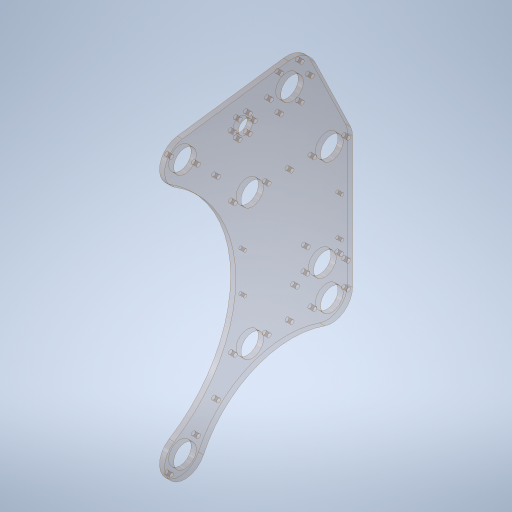
# Autodesk Inventor part: GP5-003
Saved by Autodesk Inventor 2023.4 (Build 274418000, 418)
## iProperties
Created: 2025-02-03
Part Number: GP5-003
Material: Polycarbonate, Smoke
Document SubType Name: Modeling
Designer: slick
Density: 1.2 g/cm^3
Appearance: Polycarbonate - Smoked
Mass: 361.739 g
Surface Area: 1106.19 cm^2
Volume: 301.449 cm^3
Author: slick
Autodesk Inventor part; units mm, degrees
ref_plane "YZ Plane" through (0, 0, 0) normal (1, 0, 0) x (0, 1, 0)
ref_plane "XZ Plane" through (0, 0, 0) normal (0, 1, 0) x (-1, 0, 0)
ref_plane "XY Plane" through (0, 0, 0) normal (0, 0, 1) x (1, 0, 0)
sketch "Sketch1" plane through (0, 0, 0) normal (1, 0, 0) x (0, 1, 0)
  line L0 (-12.7, 25.4) -> (12.7, 25.4) construction
  line L1 (12.7, 25.4) -> (12.7, -25.4) construction
  line L2 (12.7, -25.4) -> (-12.7, -25.4) construction
  line L3 (-12.7, -25.4) -> (-12.7, 25.4) construction
  line L4 (-12.7, 25.4) -> (12.7, -25.4) construction
  line L5 (12.7, 25.4) -> (-12.7, -25.4) construction
  circle A0 centre (-127, -49.4995) radius 38.1 construction
  circle A1 centre (-290.4981, -49.4995) radius 38.1 construction
  circle A2 centre (-127, 49.4995) radius 38.1 construction
  circle A3 centre (-290.4981, 49.4995) radius 38.1 construction
  line L6 (-127, -49.4995) -> (-127, 49.4995) construction
  line L7 (-290.4981, -49.4995) -> (-290.4981, 49.4995) construction
  line L8 (-161.925, -152.4) -> (-255.5731, -152.4) construction
  line L9 (-255.5731, -152.4) -> (-255.5731, 152.4) construction
  line L10 (-255.5731, 152.4) -> (-161.925, 152.4) construction
  line L11 (-161.925, 152.4) -> (-161.925, -152.4) construction
  line L12 (-161.925, -152.4) -> (-255.5731, 152.4) construction
  line L13 (-255.5731, -152.4) -> (-161.925, 152.4) construction
  circle A4 centre (-127, -49.4995) radius 34.925 construction
  circle A5 centre (-290.4981, -49.4995) radius 34.925 construction
  circle A6 centre (-208.749, 279.4) radius 190.5 construction
  circle A7 centre (-49.7545, 133.3399) radius 25.4 construction
  circle A8 centre (-367.7435, 133.3399) radius 25.4 construction
  circle A9 centre (-653.2508, -157.862) radius 53.975 construction
  line L14 (-596.1008, -277.7111) -> (-621.5008, -277.7111) construction
  line L15 (-621.5008, -277.7111) -> (-621.5008, -201.5111) construction
  line L16 (-621.5008, -201.5111) -> (-596.1008, -201.5111) construction
  line L17 (-596.1008, -201.5111) -> (-596.1008, -277.7111) construction
  line L18 (-596.1008, -277.7111) -> (-621.5008, -201.5111) construction
  line L19 (-621.5008, -277.7111) -> (-596.1008, -201.5111) construction
  line L20 (-685.0008, -277.7111) -> (-710.4008, -277.7111) construction
  line L21 (-710.4008, -277.7111) -> (-710.4008, -201.5111) construction
  line L22 (-710.4008, -201.5111) -> (-685.0008, -201.5111) construction
  line L23 (-685.0008, -201.5111) -> (-685.0008, -277.7111) construction
  line L24 (-685.0008, -277.7111) -> (-710.4008, -201.5111) construction
  line L25 (-710.4008, -277.7111) -> (-685.0008, -201.5111) construction
  line L26 (-498.4346, -157.862) -> (-808.067, -157.862) construction
  point P0 (0, 0)
  point P1 (-127, 0)
  point P2 (-290.4981, 0)
  point P3 (-208.749, 0)
  point P4 (-608.8008, -239.6111)
  point P5 (-697.7008, -239.6111)
  dimension "d0" = 25.4
  dimension "d1" = 50.8
  dimension "d2" = 76.2
  dimension "d4" = 98.999
  dimension "d5" = 93.6481
  dimension "d6" = 304.8
  dimension "d7" = 3.175
  dimension "d8" = 3.175
  dimension "d9" = 127
  dimension "d10" = 381
  dimension "d11" = 50.8
  dimension "d12" = 50.8
  dimension "d13" = 114.0003
  dimension "d14" = 279.4
  dimension "d35" = 49.4995
  dimension "d68" = 107.95
  dimension "d69" = 25.4
  dimension "d70" = 76.2
  dimension "d71" = 63.5
  dimension "d72" = 81.749
  dimension "d73" = 163.4981
  constraints: 54 end point, 11 midpoint, 10 centre point, 8 parallel, 7 horizontal alignment, 5 horizontal, 4 perpendicular, 4 tangent, 3 equal radius, 3 vertical alignment, 2 equal length, 2 point on circle, 2 vertical, 1 coincident
  measures "d0" distance of L1.end L2.end
  measures "d1" distance of L0.end L1.end
  measures "d2" diameter of A0
  measures "d4" distance of L6.start L6.end
  measures "d5" distance of L9.end L10.end
  measures "d6" distance of L8.end L9.end
  measures "d7" radial gap between concentric circles of A0 A4
  measures "d8" radial gap between concentric circles of A1 A5
  measures "d9" distance from line of point (0, 0) L6
  measures "d10" diameter of A6
  measures "d11" diameter of A7
  measures "d12" diameter of A8
  measures "d13" distance of L6.end A7.centre
  measures "d14" distance of A6.centre point (-208.749, 0)
  measures "d35" distance of L6.start point (-127, 0)
  measures "d68" diameter of A9
  measures "d69" distance of L15.end L16.end
  measures "d70" distance of L14.end L15.end
  measures "d71" distance of L20.start L14.end
  measures "d72" vertical distance of A9.centre point (-608.801, -239.611)
  measures "d73" distance of L7.start L6.start
sketch "Sketch2" plane through (0, 0, 0) normal (1, 0, 0) x (0, 1, 0)
  circle A0 centre (-127, -49.4995) radius 38.1 construction
  circle A1 centre (-127, 49.4995) radius 38.1 construction
  circle A2 centre (-127, -49.4995) radius 34.925 construction
  line L0 (-255.5731, 152.4) -> (-161.925, 152.4) construction
  line L1 (-161.925, -152.4) -> (-255.5731, -152.4) construction
  line L2 (-161.925, 152.4) -> (-161.925, -152.4) construction
  line L3 (-255.5731, -152.4) -> (-161.925, 152.4) construction
  line L4 (-161.925, -152.4) -> (-255.5731, 152.4) construction
  line L5 (-255.5731, -152.4) -> (-255.5731, 152.4) construction
  circle A3 centre (-290.4981, 49.4995) radius 38.1 construction
  circle A4 centre (-290.4981, -49.4995) radius 34.925 construction
  circle A5 centre (-290.4981, -49.4995) radius 38.1 construction
  line L6 (-290.4981, -49.4995) -> (-290.4981, 49.4995) construction
  line L7 (-127, -49.4995) -> (-127, 49.4995) construction
  line L8 (-12.7, -25.4) -> (-12.7, 25.4) construction
  line L9 (12.7, 25.4) -> (12.7, -25.4) construction
  line L10 (12.7, -25.4) -> (-12.7, -25.4) construction
  line L11 (-12.7, 25.4) -> (12.7, -25.4) construction
  line L12 (12.7, 25.4) -> (-12.7, -25.4) construction
  line L13 (-12.7, 25.4) -> (12.7, 25.4) construction
  circle A6 centre (-208.749, 279.4) radius 190.5 construction
  circle A7 centre (-49.7545, 133.3399) radius 25.4 construction
  circle A8 centre (-367.7435, 133.3399) radius 25.4 construction
  circle A9 centre (-127, -49.4995) radius 14.1605
  circle A10 centre (-290.4981, -49.4995) radius 14.1605
  circle A11 centre (-290.4981, 49.4995) radius 14.1605
  circle A12 centre (-127, 49.4995) radius 14.1605
  circle A13 centre (-367.7435, 133.3399) radius 14.1605
  circle A14 centre (-49.7545, 133.3399) radius 14.1605
  circle A15 centre (-38.1, 0) radius 14.1605
  circle A16 centre (-38.1, 0) radius 39.3065 construction
  circle A17 centre (-38.1, 0) radius 25.4 construction
  circle A18 centre (-38.1, 0) radius 31.75 construction
  circle A19 centre (-127, -49.4995) radius 25.781 construction
  line L14 (-127, -70.518) -> (-127, -28.481) construction
  circle A20 centre (-127, -70.518) radius 4.7625 construction
  circle A21 centre (-290.4981, -49.4995) radius 25.781 construction
  circle A22 centre (-290.4981, 49.4995) radius 25.781 construction
  circle A23 centre (-127, 49.4995) radius 25.781 construction
  line L15 (-127, -75.2805) -> (-290.4981, -75.2805)
  arc A24 (-314.7766, -40.827) -> (-378.357, 110.2636) centre (-429.0704, 0) ccw
  line L16 (-115.8012, -72.7212) -> (-24.3083, -28.5981)
  line L17 (-6.6374, 4.262) -> (-24.5844, 136.7495)
  arc A25 (-346.1366, 146.6928) -> (-71.3615, 146.6928) centre (-208.749, 231.5971) ccw
  arc A26 (-24.5844, 136.7495) -> (-71.3615, 146.6928) centre (-49.7545, 133.3399) ccw
  arc A27 (-346.1366, 146.6928) -> (-378.357, 110.2636) centre (-367.7435, 133.3399) ccw
  arc A28 (-314.7766, -40.827) -> (-290.4981, -75.2805) centre (-290.4981, -49.4995) ccw
  arc A29 (-127, -75.2805) -> (-115.8012, -72.7212) centre (-127, -49.4995) ccw
  arc A30 (-24.3083, -28.5981) -> (-6.6374, 4.262) centre (-38.1, 0) ccw
  circle A31 centre (-50.8, 58.2876) radius 19.05 construction
  circle A32 centre (-50.8, 58.2876) radius 12.7 construction
  circle A33 centre (-50.8, 58.2876) radius 8.763
  line L18 (-290.4981, 28.481) -> (-290.4981, 70.518) construction
  line L19 (-290.4981, -70.518) -> (-290.4981, -28.481) construction
  line L20 (-62.4545, 116.5921) -> (-37.0545, 150.0876) construction
  line L21 (-355.0435, 116.5921) -> (-380.4435, 150.0876) construction
  line L22 (-127, 28.481) -> (-127, 70.518) construction
  circle A34 centre (-248.1928, -40.8522) radius 14.1605
  circle A35 centre (-248.1928, -40.8522) radius 21.59 construction
  circle A36 centre (-290.4981, -49.4995) radius 21.59 construction
  line L23 (-248.1928, -61.8707) -> (-248.1928, -19.8337) construction
  point P0 (0, 0)
  point P1 (-127, 0)
  point P2 (-208.749, 0)
  point P3 (-290.4981, 0)
  point P4 (0, 0)
  point P5 (-38.1, 25.4)
  point P6 (-395.5081, 116.5261)
  point P7 (-50.8, 45.5876)
  point P8 (-39.8015, 51.9376)
  point P9 (-39.8015, 64.6376)
  point P10 (-50.8, 70.9876)
  point P11 (-61.7985, 64.6376)
  point P12 (-61.7985, 51.9376)
  dimension "d18" = 50.8
  dimension "d32" = 9.525
  dimension "d37" = 25.4
  dimension "d15" = 28.321
  dimension "d16" = 38.1
  dimension "d17" = 78.613
  dimension "d19" = 6.35
  dimension "d31" = 42.037
  dimension "d36" = 38.1
  dimension "d38" = 17.526
  dimension "d50" = 12.7
  dimension "d51" = 12.7
  dimension "d61" = 360
  dimension "d63" = 75.0595
  dimension "d64" = 76.2
  dimension "d74" = 121.5009
  dimension "d75" = 43.18
  constraints: 25 centre point, 25 coincident, 24 point on circle, 20 end point, 12 equal radius, 11 tangent, 10 vertical alignment, 7 midpoint, 6 equal length, 2 horizontal, 1 collinear, 1 horizontal alignment, 1 point on line, 14 other
  measures "d15" diameter of A9
  measures "d16" distance of A15.centre point (0, 0)
  measures "d17" diameter of A16
  measures "d31" distance of L14.end L14.start
  measures "d36" diameter of A31
  measures "d38" diameter of A33
  measures "d50" horizontal distance of point (-49.755, 133.34) L20.start
  measures "d51" horizontal distance of A8.centre L21.start
  measures "d63" distance of A7.centre A31.centre
  measures "d64" horizontal distance of L7.end A31.centre
  measures "d74" distance of A34.centre A0.centre
  measures "d75" diameter of A35
extrude "Extrusion1" add sketch "Sketch2" along normal blind 6.35
hole "Hole1" at (0, -127, -49.4995) at (0, -127, 49.4995) at (0, -161.925, 152.4) at (0, -161.925, -152.4) at (0, -255.5731, 152.4) at (0, -290.4981, 49.4995) at (0, -290.4981, -49.4995) at (0, -255.5731, -152.4) at (0, -127, -70.518) at (0, -127, -28.481) at (0, -50.8, 45.5876) at (0, -290.4981, 28.481) at (0, -290.4981, 70.518) at (0, -290.4981, -70.518) at (0, -290.4981, -28.481) at (0, -62.4545, 116.5921) at (0, -37.0545, 150.0876) at (0, -355.0435, 116.5921) at (0, -380.4435, 150.0876) at (0, -127, 28.481) at (0, -127, 70.518) at (0, -61.7985, 51.9376) at (0, -61.7985, 64.6376) at (0, -50.8, 70.9876) at (0, -39.8015, 64.6376) at (0, -39.8015, 51.9376) at (0, -248.1928, -61.8707) at (0, -248.1928, -19.8337) direction (1, 0, 0) diameter 5.1054 end through all clearance for "Flat Head Machine Screw (82)" size "#10" standard "Ansi Unified Screw Threads"
sketch "Sketch3" plane through (6.35, 0, 0) normal (1, 0, 0) x (0, 0, -1)
  circle A0 centre (0, -38.1) radius 14.1605 construction
  circle A1 centre (0, -38.1) radius 25.4 construction
  point P0 (0, 0)
  point P1 (25.4, -38.1)
  point P2 (12.7, -16.103)
  point P3 (-12.7, -16.103)
  point P4 (-25.4, -38.1)
  point P5 (-12.7, -60.097)
  point P6 (12.7, -60.097)
  dimension "d77" = 50.8
  dimension "d80" = 360
  constraints: 2 horizontal alignment, 1 coincident, 9 other
hole "Hole2" at (6.35, -38.1, -25.4) at (6.35, -16.103, -12.7) at (6.35, -16.103, 12.7) at (6.35, -38.1, 25.4) at (6.35, -60.097, 12.7) at (6.35, -60.097, -12.7) direction (-1, 0, 0) diameter 5.1054 end through all clearance for "Flat Head Machine Screw (82)" size "#10" standard "Ansi Unified Screw Threads"
sketch "Sketch4" plane through (6.35, 0, 0) normal (1, 0, 0) x (0, 0, -1)
  circle A0 centre (-12.7, -60.097) radius 2.5527 projected
  circle A1 centre (-12.7, -16.103) radius 2.5527 projected
  circle A2 centre (25.4, -38.1) radius 2.5527 projected
  circle A3 centre (12.7, -16.103) radius 2.5527 projected
  circle A4 centre (-25.4, -38.1) radius 2.5527 projected
  circle A5 centre (12.7, -60.097) radius 2.5527 projected
  circle A6 centre (61.8707, -248.1928) radius 2.5527 projected
  circle A7 centre (-64.6376, -39.8015) radius 2.5527 projected
  circle A8 centre (-64.6376, -61.7985) radius 2.5527 projected
  circle A9 centre (-70.518, -127) radius 2.5527 projected
  circle A10 centre (-150.0876, -380.4435) radius 2.5527 projected
  circle A11 centre (-150.0876, -37.0545) radius 2.5527 projected
  circle A12 centre (28.481, -290.4981) radius 2.5527 projected
  circle A13 centre (-70.518, -290.4981) radius 2.5527 projected
  circle A14 centre (-45.5876, -50.8) radius 2.5527 projected
  circle A15 centre (70.518, -127) radius 2.5527 projected
  circle A16 centre (28.481, -127) radius 2.5527 projected
  circle A17 centre (-28.481, -290.4981) radius 2.5527 projected
  circle A18 centre (70.518, -290.4981) radius 2.5527 projected
  circle A19 centre (-116.5921, -62.4545) radius 2.5527 projected
  circle A20 centre (-116.5921, -355.0435) radius 2.5527 projected
  circle A21 centre (-28.481, -127) radius 2.5527 projected
  circle A22 centre (-51.9376, -61.7985) radius 2.5527 projected
  circle A23 centre (-70.9876, -50.8) radius 2.5527 projected
  circle A24 centre (-51.9376, -39.8015) radius 2.5527 projected
  circle A25 centre (19.8337, -248.1928) radius 2.5527 projected
  arc A26 (28.5981, -24.3083) -> (-4.262, -6.6374) centre (0, -38.1) ccw projected
  line L0 (-4.262, -6.6374) -> (-136.7495, -24.5844) projected
  arc A27 (-136.7495, -24.5844) -> (-146.6928, -71.3615) centre (-133.3399, -49.7545) ccw projected
  arc A28 (-146.6928, -346.1366) -> (-146.6928, -71.3615) centre (-231.5971, -208.749) ccw projected
  arc A29 (-146.6928, -346.1366) -> (-110.2636, -378.357) centre (-133.3399, -367.7435) ccw projected
  arc A30 (40.827, -314.7766) -> (-110.2636, -378.357) centre (0, -429.0704) ccw projected
  arc A31 (40.827, -314.7766) -> (75.2805, -290.4981) centre (49.4995, -290.4981) ccw projected
  line L1 (75.2805, -290.4981) -> (75.2805, -127) projected
  arc A32 (75.2805, -127) -> (72.7212, -115.8012) centre (49.4995, -127) ccw projected
  line L2 (72.7212, -115.8012) -> (28.5981, -24.3083) projected
  circle A33 centre (-49.4995, -290.4981) radius 14.1605 projected
  circle A34 centre (-49.4995, -127) radius 14.1605 projected
  circle A35 centre (-58.2876, -50.8) radius 8.763 projected
  circle A36 centre (40.8522, -248.1928) radius 14.1605 projected
  circle A37 centre (0, -38.1) radius 14.1605 projected
  circle A38 centre (-133.3399, -49.7545) radius 14.1605 projected
  circle A39 centre (-133.3399, -367.7435) radius 14.1605 projected
  circle A40 centre (49.4995, -290.4981) radius 14.1605 projected
  circle A41 centre (49.4995, -127) radius 14.1605 projected
  circle A42 centre (-49.4995, -290.4981) radius 14.1605 projected
  line L3 (-133.3399, -367.7435) -> (-49.4995, -290.4981) construction
  line L4 (-133.3399, -49.7545) -> (-49.4995, -127) construction
  line L5 (-49.4995, -127) -> (49.4995, -127) construction
  line L6 (-49.4995, -290.4981) -> (49.4995, -290.4981) construction
  point P0 (0, 0)
  point P1 (-91.4197, -88.3773)
  point P2 (0, -127)
  point P3 (0, -290.4981)
  point P4 (-91.4197, -329.1208)
  constraints: 8 end point, 4 midpoint, 2 horizontal
hole "Hole3" at (6.35, -88.3773, 91.4197) at (6.35, -127, 0) at (6.35, -290.4981, 0) at (6.35, -329.1208, 91.4197) direction (-1, 0, 0) diameter 5.1054 end through all clearance for "Flat Head Machine Screw (82)" size "#10" standard "Ansi Unified Screw Threads"
sketch "Sketch5" plane through (0, 0, 0) normal (-1, 0, 0) x (0, 0, 1)
  line L0 (-20.2847, -219.9605) -> (-70.518, -259.5066) construction
  line L1 (-70.518, -259.5066) -> (-6.7082, -255.5595) construction
  line L2 (-6.7082, -255.5595) -> (-20.2847, -219.9605) construction
  circle A0 centre (-40.8522, -248.1928) radius 14.1605 construction
  circle A1 centre (-49.4995, -127) radius 14.1605 construction
  line L3 (-40.8522, -248.1928) -> (-49.4995, -127) construction
  line L4 (-28.6658, -247.3233) -> (-37.3131, -126.1305) construction
  line L5 (-61.6859, -127.8695) -> (-53.0386, -249.0623) construction
  arc A2 (-53.0386, -249.0623) -> (-28.6658, -247.3233) centre (-40.8522, -248.1928) ccw construction
  arc A3 (-37.3131, -126.1305) -> (-61.6859, -127.8695) centre (-49.4995, -127) ccw construction
  line L6 (-70.518, -259.5066) -> (-13.4965, -237.76) construction
  line L7 (-75.2805, -290.4981) -> (-75.2805, -127) construction
  circle A4 centre (-70.518, -259.5066) radius 4.7625 construction
  circle A5 centre (-20.2847, -219.9605) radius 4.7625 construction
  circle A6 centre (-6.7082, -255.5595) radius 4.7625 construction
  point P0 (0, 0)
  point P1 (-45.1759, -187.5964)
  dimension "d97" = 38.1
  dimension "d98" = 63.9318
  dimension "d99" = 63.9318
  dimension "d101" = 12.2174
  dimension "d102" = 31.75
  dimension "d111" = 9.525
  dimension "d112" = 9.525
  dimension "d113" = 9.525
  constraints: 16 end point, 6 coincident, 5 centre point, 5 tangent, 4 point on circle, 2 midpoint, 1 parallel, 1 point on line
  measures "d97" distance of L1.end L0.start
  measures "d98" distance of L0.end L1.end
  measures "d99" distance of L0.start L0.end
  measures "d101" radius of A3
  measures "d102" distance of L3.start L0.end
  measures "d111" diameter of A4
  measures "d112" diameter of A5
  measures "d113" diameter of A6
hole "Hole4" at (0, -248.1928, -40.8522) at (0, -259.5066, -70.518) at (0, -219.9605, -20.2847) at (0, -255.5595, -6.7082) direction (1, 0, 0) diameter 5.1054 end through all clearance for "Flat Head Machine Screw (82)" size "#10" standard "Ansi Unified Screw Threads"
sketch "Sketch6" plane through (6.35, 0, 0) normal (1, 0, 0) x (0, 0, -1)
  line L0 (62.5805, -184.1548) -> (62.5805, -233.3432) construction
  line L1 (75.2805, -290.4981) -> (75.2805, -127) construction
  circle A0 centre (20.2847, -219.9605) radius 2.5527 construction
  circle A1 centre (70.518, -259.5066) radius 2.5527 construction
  circle A2 centre (6.7082, -255.5595) radius 2.5527 construction
  circle A3 centre (0, -290.4981) radius 2.5527 construction
  circle A4 centre (-91.4197, -88.3773) radius 2.5527 construction
  circle A5 centre (0, -127) radius 2.5527 construction
  circle A6 centre (-91.4197, -329.1208) radius 2.5527 construction
  circle A7 centre (-12.7, -60.097) radius 2.5527 construction
  circle A8 centre (-12.7, -16.103) radius 2.5527 construction
  circle A9 centre (25.4, -38.1) radius 2.5527 construction
  circle A10 centre (12.7, -16.103) radius 2.5527 construction
  circle A11 centre (-25.4, -38.1) radius 2.5527 construction
  circle A12 centre (12.7, -60.097) radius 2.5527 construction
  circle A13 centre (61.8707, -248.1928) radius 2.5527 construction
  circle A14 centre (-64.6376, -39.8015) radius 2.5527 construction
  circle A15 centre (-64.6376, -61.7985) radius 2.5527 construction
  circle A16 centre (-70.518, -127) radius 2.5527 construction
  circle A17 centre (-150.0876, -380.4435) radius 2.5527 construction
  circle A18 centre (-150.0876, -37.0545) radius 2.5527 construction
  circle A19 centre (28.481, -290.4981) radius 2.5527 construction
  circle A20 centre (-70.518, -290.4981) radius 2.5527 construction
  circle A21 centre (-45.5876, -50.8) radius 2.5527 construction
  circle A22 centre (70.518, -127) radius 2.5527 construction
  circle A23 centre (28.481, -127) radius 2.5527 construction
  circle A24 centre (-28.481, -290.4981) radius 2.5527 construction
  circle A25 centre (70.518, -290.4981) radius 2.5527 construction
  circle A26 centre (-116.5921, -62.4545) radius 2.5527 construction
  circle A27 centre (-116.5921, -355.0435) radius 2.5527 construction
  circle A28 centre (-28.481, -127) radius 2.5527 construction
  circle A29 centre (-51.9376, -61.7985) radius 2.5527 construction
  circle A30 centre (-70.9876, -50.8) radius 2.5527 construction
  circle A31 centre (-51.9376, -39.8015) radius 2.5527 construction
  circle A32 centre (19.8337, -248.1928) radius 2.5527 construction
  circle A33 centre (49.4995, -127) radius 14.1605 construction
  circle A34 centre (49.4995, -290.4981) radius 14.1605 construction
  circle A35 centre (-133.3399, -367.7435) radius 14.1605 construction
  circle A36 centre (-133.3399, -49.7545) radius 14.1605 construction
  circle A37 centre (0, -38.1) radius 14.1605 construction
  circle A38 centre (40.8522, -248.1928) radius 14.1605 construction
  circle A39 centre (-58.2876, -50.8) radius 8.763 construction
  circle A40 centre (-49.4995, -127) radius 14.1605 construction
  circle A41 centre (-49.4995, -290.4981) radius 14.1605 construction
  line L2 (28.5981, -24.3083) -> (72.7212, -115.8012) construction
  arc A42 (75.2805, -127) -> (72.7212, -115.8012) centre (49.4995, -127) ccw construction
  line L3 (75.2805, -127) -> (75.2805, -290.4981) construction
  arc A43 (40.827, -314.7766) -> (75.2805, -290.4981) centre (49.4995, -290.4981) ccw construction
  arc A44 (40.827, -314.7766) -> (-110.2636, -378.357) centre (0, -429.0704) ccw construction
  arc A45 (-146.6928, -346.1366) -> (-110.2636, -378.357) centre (-133.3399, -367.7435) ccw construction
  arc A46 (-146.6928, -346.1366) -> (-146.6928, -71.3615) centre (-231.5971, -208.749) ccw construction
  arc A47 (-136.7495, -24.5844) -> (-146.6928, -71.3615) centre (-133.3399, -49.7545) ccw construction
  line L4 (-136.7495, -24.5844) -> (-4.262, -6.6374) construction
  arc A48 (28.5981, -24.3083) -> (-4.262, -6.6374) centre (0, -38.1) ccw construction
  line L5 (49.4995, -127) -> (49.4995, -290.4981) construction
  line L6 (-58.0695, -184.1548) -> (-58.0695, -233.3432) construction
  point P0 (0, 0)
  point P1 (49.4995, -208.749)
  point P2 (62.5805, -208.749)
  point P3 (-58.0695, -208.749)
  dimension "d114" = 49.1884
  dimension "d115" = 12.7
  dimension "d116" = 49.1884
  dimension "d117" = 120.65
  constraints: 6 end point, 4 coincident, 3 midpoint, 3 vertical, 2 horizontal alignment
  measures "d114" distance of L0.start L0.end
  measures "d115" distance between parallel lines of L1 L0
  measures "d116" distance of L6.start L6.end
  measures "d117" distance of point (62.581, -208.749) point (-58.069, -208.749)
hole "Hole5" at (6.35, -184.1548, 58.0695) at (6.35, -233.3432, 58.0695) at (6.35, -233.3432, -62.5805) at (6.35, -184.1548, -62.5805) direction (-1, 0, 0) diameter 3.81 end through all clearance for "Flat Head Machine Screw (82)" size "#6" standard "Ansi Unified Screw Threads"
equation "\"d73\" = 2 * d72"
equation "\"d51\" = d50"
equation "\"d99\" = d98"
body "Solid1"
